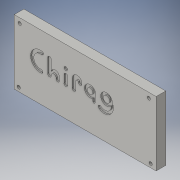
# Autodesk Inventor part: NameTag
Saved by Autodesk Inventor 2016 (Build 200138000, 138)
## iProperties
Created: 2016-09-22
Part Number: NameTag
Material: Generic
Document SubType Name: Modeling
Designer: Shaan Sharma
Density: 1 g/cm^3
Appearance: Default
Author: Shaan Sharma
Autodesk Inventor part; units mm, degrees
ref_plane "YZ Plane" through (0, 0, 0) normal (1, 0, 0) x (0, 1, 0)
ref_plane "XZ Plane" through (0, 0, 0) normal (0, 1, 0) x (-1, 0, 0)
ref_plane "XY Plane" through (0, 0, 0) normal (0, 0, 1) x (1, 0, 0)
sketch "Sketch1" plane through (0, 0, 0) normal (0, 0, 1) x (1, 0, 0)
  line L0 (-127, 50.8) -> (152.4, 50.8)
  line L1 (152.4, 50.8) -> (152.4, -76.2)
  line L2 (152.4, -76.2) -> (-127, -76.2)
  line L3 (-127, -76.2) -> (-127, 50.8)
  point P0 (0, 0)
  dimension "d0" = 127
  dimension "d1" = 279.4
  constraints: 8 end point, 2 parallel, 1 horizontal, 1 perpendicular
  measures "d0" distance of L2.end L0.start
  measures "d1" distance of L1.end L2.end
extrude "Extrusion1" add sketch "Sketch1" along normal blind 19.05
sketch "Sketch2" plane through (0, 0, 19.05) normal (0, 0, 1) x (1, 0, 0)
  arc A0 (-73.0244, 15.878) -> (-73.0246, -22.228) centre (-75.5284, -3.175) ccw
  arc A1 (-73.1475, 9.5485) -> (-73.025, -15.875) centre (-75.5284, -3.175) ccw
  arc A2 (-73.1475, 9.5485) -> (-73.0244, 15.878) centre (-72.5572, 12.703) ccw
  arc A3 (-73.2146, -22.252) -> (-73.025, -15.875) centre (-73.603, -19.0491) ccw
  line L0 (-61.1063, -15.875) -> (-61.1063, 9.5485)
  arc A4 (-61.1063, -15.875) -> (-53.975, -15.875) centre (-57.5407, -16.9375) ccw
  arc A5 (-53.975, 9.5485) -> (-61.1063, 9.5485) centre (-57.5407, 10.5766) ccw
  line L1 (-53.975, 9.5485) -> (-53.975, -9.525)
  arc A6 (-38.1, -9.525) -> (-53.975, -9.525) centre (-46.0375, -11.2959) ccw
  line L2 (-38.1, -9.525) -> (-38.1, -17.8441)
  arc A7 (-44.6048, -17.106) -> (-38.1, -17.8441) centre (-41.3943, -17.8441) ccw
  arc A8 (-44.6048, -17.106) -> (-53.975, -15.875) centre (-49.231, -16.0424) ccw
  circle A9 centre (-25.4, 9.5485) radius 3.4758
  arc A10 (-28.8758, -16.0424) -> (-21.9242, -16.0424) centre (-25.4, -17.3897) ccw
  arc A11 (-21.9242, -3.1632) -> (-28.8758, -3.1632) centre (-25.4, -2.0594) ccw
  line L3 (-28.8758, -3.1632) -> (-28.8758, -16.0424)
  line L4 (-21.9242, -3.1632) -> (-21.9242, -16.0424)
  arc A12 (-12.6126, -16.1823) -> (-6.2626, -16.1823) centre (-9.4376, -17.7266) ccw
  line L5 (-12.6126, -16.1823) -> (-12.6126, -0.1511)
  arc A13 (6.1684, -2.399) -> (-12.6126, -0.1511) centre (-3.0876, -0.1511) ccw
  line L6 (-6.2626, -16.1823) -> (-6.2626, -6.4899)
  arc A14 (0, 0) -> (6.1684, -2.399) centre (2.9241, -1.6111) ccw
  arc A15 (0, 0) -> (-6.2626, -6.4899) centre (-2.3813, -3.9688) ccw
  circle A16 centre (22.4437, -5.0591) radius 11.2637
  circle A17 centre (22.4437, -5.0591) radius 5.6341
  line L7 (28.0778, -14.8125) -> (28.0778, -19.8605)
  line L8 (32.1971, -10.6931) -> (32.1971, -19.8605)
  arc A18 (28.0778, -19.8605) -> (32.1971, -19.8605) centre (30.1375, -19.8605) ccw
  circle A19 centre (54.7585, -2.6676) radius 11.4369
  circle A20 centre (54.7585, -2.6676) radius 6.4193
  arc A21 (43.3216, -19.5287) -> (64.2241, -9.0869) centre (51.9093, -10.5775) ccw
  arc A22 (43.3216, -19.5287) -> (40.471, -26.1835) centre (41.8963, -22.8561) ccw
  arc A23 (40.471, -26.1835) -> (66.1955, -2.6676) centre (50.4992, -11.3254) ccw
  constraints: 43 point on circle, 24 centre point, 18 end point, 8 tangent, 8 vertical, 2 coincident, 1 concentric, 1 parallel
emboss "Emboss1" sketch "Sketch2" operation cut depth 2.54 direction (0, 0, -1)
hole "Hole1" at (-116.218, 41.2565, 19.05) direction (0, 0, -1) diameter 6.35 end through all
hole "Hole2" at (-118.0348, -68.3727, 19.05) direction (0, 0, -1) diameter 6.35 end through all
hole "Hole3" at (138.1431, 40.9115, 19.05) direction (0, 0, -1) diameter 6.35 end through all
hole "Hole4" at (141.7768, -68.7579, 19.05) direction (0, 0, -1) diameter 6.35 end through all
body "Solid1"
